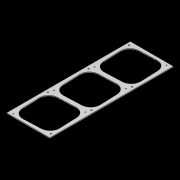
# Autodesk Inventor part: top_140mm
Saved by Autodesk Inventor 2018 (Build 220112000, 112)
## iProperties
Created: 2020-10-17
Part Number: top_140mm
Material: アルミニウム 6061
Document SubType Name: Modeling
Designer: gisen
Density: 2.7 g/cm^3
Appearance: アルミニウム - フラット
Author: gisen
Autodesk Inventor part; units mm, degrees
ref_plane "YZ Plane" through (0, 0, 0) normal (1, 0, 0) x (0, 1, 0)
ref_plane "XZ Plane" through (0, 0, 0) normal (0, 1, 0) x (-1, 0, 0)
ref_plane "XY Plane" through (0, 0, 0) normal (0, 0, 1) x (1, 0, 0)
sketch "スケッチ1" plane through (0, 0, 0) normal (0, 0, 1) x (1, 0, 0)
  line L0 (-75, -215) -> (75, -215)
  line L1 (75, -215) -> (75, 215)
  line L2 (75, 215) -> (-75, 215)
  line L3 (-75, 215) -> (-75, -215)
  line L4 (-75, -215) -> (75, 215) construction
  line L5 (75, -215) -> (-75, 215) construction
  line L6 (-65, -215) -> (-65, 215) construction
  line L7 (-65, 59.8957) -> (59.8957, 65) construction
  line L8 (59.8957, 65) -> (65, -59.8957) construction
  line L9 (65, -59.8957) -> (-59.8957, -65) construction
  line L10 (-59.8957, -65) -> (-65, 59.8957) construction
  line L11 (-65, 59.8957) -> (65, -59.8957) construction
  line L12 (59.8957, 65) -> (-59.8957, -65) construction
  circle A0 centre (-65, 59.8957) radius 2.25
  line L13 (-67.0832, -72.8) -> (72.8, -67.0832) construction
  line L14 (72.8, -67.0832) -> (67.0832, 72.8) construction
  line L15 (67.0832, 72.8) -> (-72.8, 67.0832) construction
  line L16 (-72.8, 67.0832) -> (-67.0832, -72.8) construction
  line L17 (-67.0832, -72.8) -> (67.0832, 72.8) construction
  line L18 (72.8, -67.0832) -> (-72.8, 67.0832) construction
  line L19 (0, 0) -> (0, 70.0584) construction
  circle A1 centre (65, -59.8957) radius 2.25
  circle A2 centre (59.8957, 65) radius 1.6
  circle A3 centre (-59.8957, -65) radius 1.6
  line L20 (-63.6933, 27.9224) -> (-61.2024, -33.0267)
  line L21 (-27.9224, -63.6933) -> (33.0267, -61.2024)
  line L22 (63.6933, -27.9224) -> (61.2024, 33.0267)
  line L23 (27.9224, 63.6933) -> (-33.0267, 61.2024)
  line L24 (-62.4479, -2.5521) -> (62.4479, 2.5521) construction
  arc A4 (-33.0267, 61.2024) -> (-63.6933, 27.9224) centre (-31.72, 29.2291) ccw
  arc A5 (61.2024, 33.0267) -> (27.9224, 63.6933) centre (29.2291, 31.72) ccw
  arc A6 (33.0267, -61.2024) -> (63.6933, -27.9224) centre (31.72, -29.2291) ccw
  arc A7 (-61.2024, -33.0267) -> (-27.9224, -63.6933) centre (-29.2291, -31.72) ccw
  circle A8 centre (-65, -81.1043) radius 2.25
  circle A9 centre (-59.8957, -206) radius 1.6
  circle A10 centre (65, -200.8957) radius 2.25
  circle A11 centre (59.8957, -76) radius 1.6
  arc A12 (61.2024, -107.9733) -> (27.9224, -77.3067) centre (29.2291, -109.28) ccw
  line L25 (27.9224, -77.3067) -> (-33.0267, -79.7976)
  arc A13 (-33.0267, -79.7976) -> (-63.6933, -113.0776) centre (-31.72, -111.7709) ccw
  line L26 (-63.6933, -113.0776) -> (-61.2024, -174.0267)
  arc A14 (-61.2024, -174.0267) -> (-27.9224, -204.6933) centre (-29.2291, -172.72) ccw
  line L27 (-27.9224, -204.6933) -> (33.0267, -202.2024)
  arc A15 (33.0267, -202.2024) -> (63.6933, -168.9224) centre (31.72, -170.2291) ccw
  line L28 (63.6933, -168.9224) -> (61.2024, -107.9733)
  circle A16 centre (-65, 200.8957) radius 2.25
  circle A17 centre (-59.8957, 76) radius 1.6
  circle A18 centre (65, 81.1043) radius 2.25
  circle A19 centre (59.8957, 206) radius 1.6
  arc A20 (61.2024, 174.0267) -> (27.9224, 204.6933) centre (29.2291, 172.72) ccw
  line L29 (27.9224, 204.6933) -> (-33.0267, 202.2024)
  arc A21 (-33.0267, 202.2024) -> (-63.6933, 168.9224) centre (-31.72, 170.2291) ccw
  line L30 (-63.6933, 168.9224) -> (-61.2024, 107.9733)
  arc A22 (-61.2024, 107.9733) -> (-27.9224, 77.3067) centre (-29.2291, 109.28) ccw
  line L31 (-27.9224, 77.3067) -> (33.0267, 79.7976)
  arc A23 (33.0267, 79.7976) -> (63.6933, 113.0776) centre (31.72, 111.7709) ccw
  line L32 (63.6933, 113.0776) -> (61.2024, 174.0267)
  circle A24 centre (-65, 59.8957) radius 2.25
  circle A25 centre (-59.8957, -65) radius 1.6
  circle A26 centre (65, -59.8957) radius 2.25
  circle A27 centre (59.8957, 65) radius 1.6
  arc A28 (61.2024, 33.0267) -> (27.9224, 63.6933) centre (29.2291, 31.72) ccw
  line L33 (27.9224, 63.6933) -> (-33.0267, 61.2024)
  arc A29 (-33.0267, 61.2024) -> (-63.6933, 27.9224) centre (-31.72, 29.2291) ccw
  line L34 (-63.6933, 27.9224) -> (-61.2024, -33.0267)
  arc A30 (-61.2024, -33.0267) -> (-27.9224, -63.6933) centre (-29.2291, -31.72) ccw
  line L35 (-27.9224, -63.6933) -> (33.0267, -61.2024)
  arc A31 (33.0267, -61.2024) -> (63.6933, -27.9224) centre (31.72, -29.2291) ccw
  line L36 (63.6933, -27.9224) -> (61.2024, 33.0267)
  point P0 (-65, 59.8957)
  point P1 (59.8957, 65)
  point P2 (-65, -81.1043)
  point P3 (59.8957, -76)
  point P4 (-62.4479, -143.5521)
  point P5 (62.4479, -138.4479)
  point P6 (-65, 200.8957)
  point P7 (59.8957, 206)
  point P8 (-62.4479, 138.4479)
  point P9 (62.4479, 143.5521)
  point P10 (-65, 59.8957)
  point P11 (59.8957, 65)
  dimension "d0" = 150
  dimension "d1" = 430
  dimension "d3" = 65
  dimension "d4" = 125
  dimension "d7" = 4.5
  dimension "d8" = 140
  dimension "d9" = 70.0584
  dimension "d10" = 3.2
  dimension "d24" = 125
  dimension "d25" = 32
  dimension "d28" = 141
  dimension "d31" = 141
  constraints: 74 end point, 32 centre point, 32 point on circle, 20 point on line, 10 midpoint, 9 parallel, 8 perpendicular, 8 tangent, 5 equal radius, 4 coincident, 3 vertical, 1 collinear, 1 horizontal, 96 other
  measures "d0" distance of L2.end L1.end
  measures "d1" distance of L1.end L0.end
  measures "d3" distance from line of L19.start L6
  measures "d4" distance of L7.end L8.end
  measures "d7" diameter of A0
  measures "d8" distance of L14.end L13.end
  measures "d9" distance of L19.start L19.end
  measures "d10" diameter of A2
  measures "d24" distance of point (59.896, 65) point (-65, 59.896)
  measures "d25" radius of A4
  measures "d28" distance of A0.centre A8.centre
  measures "d31" distance of A0.centre A16.centre
extrude "押し出し1" add sketch "スケッチ1" along normal blind 3
fillet "フィレット1" [suppressed]
sketch "スケッチ3" plane through (0, 0, 3) normal (0, 0, 1) x (1, 0, 0)
  line L0 (-75, -215) -> (75, -215) construction
  line L1 (75, 215) -> (-75, 215) construction
  line L2 (-75, 215) -> (75, 215)
  line L3 (75, 215) -> (75, 235)
  line L4 (75, 235) -> (-75, 235)
  line L5 (-75, 235) -> (-75, 215)
  line L6 (-75, -215) -> (75, -215)
  line L7 (75, -215) -> (75, -255)
  line L8 (75, -255) -> (-75, -255)
  line L9 (-75, -255) -> (-75, -215)
  circle A0 centre (-65, 225) radius 2.15
  circle A1 centre (65, 225) radius 2.15
  circle A2 centre (-65, -245) radius 2.15
  circle A3 centre (65, -245) radius 2.15
  point P0 (0, 0)
  dimension "d34" = 40
  dimension "d35" = 20
  dimension "d36" = 4.3
  dimension "d37" = 10
  dimension "d38" = 10
  dimension "d39" = 10
  dimension "d40" = 10
  constraints: 16 end point, 4 centre point, 4 parallel, 3 equal radius, 2 horizontal, 2 horizontal alignment, 2 perpendicular, 2 vertical alignment
  measures "d34" distance of L0.end L7.end
  measures "d35" distance of L1.start L3.end
  measures "d36" diameter of A0
  measures "d37" distance from line of L5 A0.centre
  measures "d38" distance from line of L3 A1.centre
  measures "d39" distance from line of L4 A0.centre
  measures "d40" distance from line of L8 A3.centre
extrude "押し出し2" [suppressed]
equation "\"d38\" = d37"
